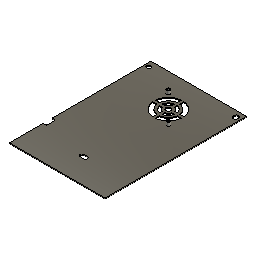
Ender 3 mainboard cover no-fan v10 (Autodesk Fusion 360 design; units mm, degrees)
Autodesk Fusion 360 part; units mm, degrees
sketch "Sketch1" plane through (0, 0, 0) normal (0, 0, 1) x (1, 0, 0)
  line L0 (-57.2, 86.75) -> (56, 86.75)
  line L1 (56, 86.75) -> (56, -80.25)
  line L2 (56, -80.25) -> (-57.2, -80.25)
  line L3 (-57.2, -80.25) -> (-57.2, 86.75)
  circle A0 centre (-52.2, 79.25) radius 2
  line L4 (48, 80) -> (48, 78.5)
  arc A1 (48, 78.5) -> (52, 78.5) centre (50, 78.5) ccw
  line L5 (52, 78.5) -> (52, 80)
  arc A2 (52, 80) -> (48, 80) centre (50, 80) ccw
  line L6 (50, 80) -> (50, 78.5) construction
  line L7 (-1.25, -51.95) -> (2.95, -51.95)
  arc A3 (2.95, -51.95) -> (2.95, -48.45) centre (2.95, -50.2) ccw
  line L8 (2.95, -48.45) -> (-1.25, -48.45)
  arc A4 (-1.25, -48.45) -> (-1.25, -51.95) centre (-1.25, -50.2) ccw
  line L9 (-3, -50.2) -> (4.7, -50.2) construction
  line L10 (-57.2, -30.05) -> (-53.2, -30.05)
  line L11 (-53.2, -30.05) -> (-53.2, -39.95)
  line L12 (-53.2, -39.95) -> (-57.2, -39.95)
  line L13 (-57.2, -39.95) -> (-57.2, -30.05)
  dimension "d1" = 113.2
  dimension "d2" = 167
  dimension "d3" = 4
  dimension "d4" = 5
  dimension "d5" = 7.5
  dimension "d6" = 4
  dimension "d7" = 1.5
  dimension "d8" = 6
  dimension "d9" = 6.75
  dimension "d10" = 3.5
  dimension "d11" = 7.7
  dimension "d12" = 28.3
  dimension "d13" = 51.3
  dimension "d14" = 9.9
  dimension "d15" = 4
  dimension "d16" = 40.3
  constraint horizontal L0
  constraint vertical L1
  constraint horizontal L2
  constraint vertical L3
  constraint tangent L4 A1
  constraint tangent A1 L5
  constraint parallel L4 L5
  constraint tangent L5 A2
  constraint tangent L4 A2
  constraint vertical L6
  constraint tangent L7 A3
  constraint tangent A3 L8
  constraint parallel L7 L8
  constraint tangent L8 A4
  constraint tangent L7 A4
  constraint midpoint A4 L9.start
  constraint midpoint A3 L9.end
  constraint horizontal L9
  constraint horizontal L10
  constraint vertical L11
  constraint horizontal L12
  constraint vertical L13
  constraint coincident L3 L10.start
  measures "d1" distance of L0.start L0.end
  measures "d2" distance of L0.start L2.end
  measures "d3" diameter of A0
  measures "d4" distance of L3 A0.centre
  measures "d5" distance of L0 A0.centre
  measures "d6" diameter of A1
  measures "d7" distance of A2.centre A1.centre
  measures "d8" distance of L1 A1.centre
  measures "d9" distance of L0 A2.centre
  measures "d10" diameter of A3
  measures "d11" distance of L9.start L9.end
  measures "d12" distance of L2 L7
  measures "d13" distance of L1 L9.end
  measures "d14" distance of L10.start L12.end
  measures "d15" distance of L10.start L10.end
  measures "d16" distance of L2 L12
  measures "d47" distance of L0.start
extrude "Extrude1" add sketch "Sketch1" along normal blind 1 contours L0 L1 L2 L3 L10 L11 L12
sketch "Sketch4" plane through (0, 0, 1) normal (0, 0, 1) x (-1, 0, 0)
  arc A0 (-52, -80) -> (-48, -80) centre (-50, -80) ccw
  line L0 (-52, -80) -> (-52, -78.5)
  arc A1 (-48, -78.5) -> (-52, -78.5) centre (-50, -78.5) ccw
  line L1 (-48, -78.5) -> (-48, -80)
  arc A2 (1.25, 48.45) -> (1.25, 51.95) centre (1.25, 50.2) ccw
  line L2 (1.25, 48.45) -> (-2.95, 48.45)
  arc A3 (-2.95, 51.95) -> (-2.95, 48.45) centre (-2.95, 50.2) ccw
  line L3 (-2.95, 51.95) -> (1.25, 51.95)
  circle A4 centre (52.2, -79.25) radius 2
  line L4 (57.2, 30.05) -> (53.2, 30.05)
  line L5 (53.2, 30.05) -> (53.2, 39.95)
  line L6 (53.2, 39.95) -> (57.2, 39.95)
  line L7 (57.2, 39.95) -> (57.2, 80.25)
  line L8 (57.2, 80.25) -> (-56, 80.25)
  line L9 (-56, 80.25) -> (-56, -86.75)
  line L10 (-56, -86.75) -> (57.2, -86.75)
  line L11 (57.2, -86.75) -> (57.2, 30.05)
  circle A5 centre (-2.375, -47.675) radius 16.875
  circle A6 centre (-2.375, -47.675) radius 12
  circle A7 centre (-2.375, -47.675) radius 9
  circle A8 centre (-2.375, -47.675) radius 6
  circle A9 centre (-2.375, -47.675) radius 3
  line L12 (-3.875, -66.4009) -> (-0.875, -66.4009)
  line L13 (-0.875, -66.4009) -> (-0.875, -28.9491)
  line L14 (-0.875, -28.9491) -> (-3.875, -28.9491)
  line L15 (-3.875, -28.9491) -> (-3.875, -66.4009)
  line L16 (-3.875, -66.4009) -> (-0.875, -28.9491) construction
  line L17 (-0.875, -66.4009) -> (-3.875, -28.9491) construction
  line L18 (-24.5082, -46.175) -> (19.7582, -46.175)
  line L19 (19.7582, -46.175) -> (19.7582, -49.175)
  line L20 (19.7582, -49.175) -> (-24.5082, -49.175)
  line L21 (-24.5082, -49.175) -> (-24.5082, -46.175)
  line L22 (-24.5082, -46.175) -> (19.7582, -49.175) construction
  line L23 (19.7582, -46.175) -> (-24.5082, -49.175) construction
  point P0 (-2.375, -47.675)
  point P1 (-2.375, -47.675)
  dimension "d42" = 33.75
  dimension "d43" = 24
  dimension "d44" = 18
  dimension "d45" = 12
  dimension "d46" = 6
  dimension "d47" = 3
  dimension "d48" = 3
  dimension "d59" = 39.075
  dimension "d60" = 53.625
  constraint concentric A5 A6
  constraint concentric A5 A7
  constraint concentric A6 A8
  constraint concentric A8 A9
  constraint perpendicular L12 L13
  constraint parallel L12 L14
  constraint parallel L13 L15
  constraint horizontal L12
  constraint coincident L16 P1
  constraint coincident L17 P1
  constraint coincident P1 P0
  constraint perpendicular L18 L19
  constraint parallel L18 L20
  constraint parallel L19 L21
  constraint horizontal L18
  constraint coincident L22 P1
  constraint coincident L23 P1
  measures "d42" diameter of A5
  measures "d43" diameter of A6
  measures "d44" diameter of A7
  measures "d45" diameter of A8
  measures "d46" diameter of A9
  measures "d47" distance of L13.end L14.end
  measures "d48" distance of L18.end L19.end
  measures "d59" distance of L10 P1
  measures "d60" distance of L9 P1
extrude "Extrude4" cut sketch "Sketch4" against normal through all contours A5 A6 L13 L18 | A5 A6 L13 L20 | A5 A6 L15 L18 | A7 A8 L13 L18 | A5 A6 L15 L20 | A7 A8 L13 L20 | A7 A8 L15 L18 | A9 L13 L18 | A9 L13 L18 L20 | A7 A8 L15 L20 | A9 L13 L20 | A9 L13 L15 L18 | L13 L15 L18 L20 | A9 L13 L15 L20 | A9 L15 L18 | A9 L15 L18 L20 | A9 L15 L20
sketch "Sketch5" plane through (0, 0, 1) normal (0, 0, 1) x (-1, 0, 0)
  arc A0 (-0.875, -59.5809) -> (9.5309, -49.175) centre (-2.375, -47.675) ccw
  line L0 (9.5309, -49.175) -> (14.4332, -49.175)
  arc A1 (-0.875, -64.4832) -> (14.4332, -49.175) centre (-2.375, -47.675) ccw
  line L1 (-0.875, -64.4832) -> (-0.875, -59.5809)
  arc A2 (-14.2809, -49.175) -> (-3.875, -59.5809) centre (-2.375, -47.675) ccw
  line L2 (-3.875, -59.5809) -> (-3.875, -64.4832)
  arc A3 (-19.1832, -49.175) -> (-3.875, -64.4832) centre (-2.375, -47.675) ccw
  line L3 (-19.1832, -49.175) -> (-14.2809, -49.175)
  arc A4 (-3.875, -35.7691) -> (-14.2809, -46.175) centre (-2.375, -47.675) ccw
  line L4 (-14.2809, -46.175) -> (-19.1832, -46.175)
  arc A5 (-3.875, -30.8668) -> (-19.1832, -46.175) centre (-2.375, -47.675) ccw
  line L5 (-3.875, -30.8668) -> (-3.875, -35.7691)
  arc A6 (-0.875, -53.4845) -> (3.4345, -49.175) centre (-2.375, -47.675) ccw
  line L6 (3.4345, -49.175) -> (6.4991, -49.175)
  arc A7 (-0.875, -56.5491) -> (6.4991, -49.175) centre (-2.375, -47.675) ccw
  line L7 (-0.875, -56.5491) -> (-0.875, -53.4845)
  arc A8 (-3.875, -41.8655) -> (-8.1845, -46.175) centre (-2.375, -47.675) ccw
  line L8 (-8.1845, -46.175) -> (-11.2491, -46.175)
  arc A9 (-3.875, -38.8009) -> (-11.2491, -46.175) centre (-2.375, -47.675) ccw
  line L9 (-3.875, -38.8009) -> (-3.875, -41.8655)
  arc A10 (3.4345, -46.175) -> (-0.875, -41.8655) centre (-2.375, -47.675) ccw
  line L10 (-0.875, -41.8655) -> (-0.875, -38.8009)
  arc A11 (6.4991, -46.175) -> (-0.875, -38.8009) centre (-2.375, -47.675) ccw
  line L11 (6.4991, -46.175) -> (3.4345, -46.175)
  circle A12 centre (-2.375, -47.675) radius 3
  arc A13 (9.5309, -46.175) -> (-0.875, -35.7691) centre (-2.375, -47.675) ccw
  line L12 (-0.875, -35.7691) -> (-0.875, -30.8668)
  arc A14 (14.4332, -46.175) -> (-0.875, -30.8668) centre (-2.375, -47.675) ccw
  line L13 (14.4332, -46.175) -> (9.5309, -46.175)
  arc A15 (-8.1845, -49.175) -> (-3.875, -53.4845) centre (-2.375, -47.675) ccw
  line L14 (-3.875, -53.4845) -> (-3.875, -56.5491)
  arc A16 (-11.2491, -49.175) -> (-3.875, -56.5491) centre (-2.375, -47.675) ccw
  line L15 (-11.2491, -49.175) -> (-8.1845, -49.175)
  arc A17 (-52, -80) -> (-48, -80) centre (-50, -80) ccw
  line L16 (-52, -80) -> (-52, -78.5)
  arc A18 (-48, -78.5) -> (-52, -78.5) centre (-50, -78.5) ccw
  line L17 (-48, -78.5) -> (-48, -80)
  arc A19 (1.25, 48.45) -> (1.25, 51.95) centre (1.25, 50.2) ccw
  line L18 (1.25, 48.45) -> (-2.95, 48.45)
  arc A20 (-2.95, 51.95) -> (-2.95, 48.45) centre (-2.95, 50.2) ccw
  line L19 (-2.95, 51.95) -> (1.25, 51.95)
  circle A21 centre (52.2, -79.25) radius 2
  line L20 (57.2, 30.05) -> (53.2, 30.05)
  line L21 (53.2, 30.05) -> (53.2, 39.95)
  line L22 (53.2, 39.95) -> (57.2, 39.95)
  line L23 (57.2, 39.95) -> (57.2, 80.25)
  line L24 (57.2, 80.25) -> (-56, 80.25)
  line L25 (-56, 80.25) -> (-56, -86.75)
  line L26 (-56, -86.75) -> (57.2, -86.75)
  line L27 (57.2, -86.75) -> (57.2, 30.05)
  circle A22 centre (13.6056, -63.6556) radius 2.05
  circle A23 centre (-18.3556, -31.6944) radius 2.05
  line L28 (13.6056, -63.6556) -> (-18.3556, -31.6944) construction
  circle A24 centre (13.6056, -63.6556) radius 1.25
  circle A25 centre (-18.3556, -31.6944) radius 1.25
  dimension "d51" = 4.1
  dimension "d52" = 4.1
  dimension "d53" = 45.2
  dimension "d54" = 45
  dimension "d55" = 2.5
  dimension "d56" = 2.5
  constraint coincident A22.centre L28.start
  constraint coincident A23.centre L28.end
  constraint coincident A0.centre L28
  constraint midpoint A0.centre L28
  measures "d51" diameter of A22
  measures "d52" diameter of A23
  measures "d53" distance of A22.centre A23.centre
  measures "d54" angle of L4 L28
  measures "d55" diameter of A24
  measures "d56" diameter of A25
extrude "Extrude5" add sketch "Sketch5" along normal blind 4.2 contours A22 | A23
fillet "Fillet4" radius 1 8 edges at (56, -80.25, 0.5) (-57.2, -80.25, 0.5) (-57.2, -39.95, 0.5) (-53.2, -39.95, 0.5) (-57.2, -30.05, 0.5) (-53.2, -30.05, 0.5) (-57.2, 86.75, 0.5) (56, 86.75, 0.5)
fillet "Fillet5" radius 0.5 50 edges at (-56.9071, -79.9571, 1) (-0.6, -80.25, 1) (55.7071, -79.9571, 1) (56, 3.25, 1) (55.7071, 86.4571, 1) (-0.6, 86.75, 1) (-56.9071, 86.4571, 1) (-57.2, 28.35, 1) (-56.9071, -29.7571, 1) (-55.2, -30.05, 1) (-53.4929, -30.3429, 1) (-53.2, -35, 1) (-53.4929, -39.6571, 1) (-55.2, -39.95, 1) (-56.9071, -40.2429, 1) (-57.2, -60.1, 1) (-56.9071, -40.2429, 0) (-55.2, -39.95, 0) (-53.4929, -39.6571, 0) (-53.2, -35, 0) (-53.4929, -30.3429, 0) (-55.2, -30.05, 0) (-56.9071, -29.7571, 0) (-57.2, 28.35, 0) (-56.9071, 86.4571, 0) (-0.6, 86.75, 0) (55.7071, 86.4571, 0) (56, 3.25, 0) (55.7071, -79.9571, 0) (-0.6, -80.25, 0) (-56.9071, -79.9571, 0) (-57.2, -60.1, 0) (-3, -50.2, 1) (0.85, -48.45, 1) (4.7, -50.2, 1) (0.85, -51.95, 1) (-3, -50.2, 0) (0.85, -48.45, 0) (4.7, -50.2, 0) (0.85, -51.95, 0) (-54.0647, 79.9732, 1) (-54.0647, 79.9732, 0) (50, 82, 1) (52, 79.25, 1) (50, 76.5, 1) (48, 79.25, 1) (50, 82, 0) (52, 79.25, 0) (50, 76.5, 0) (48, 79.25, 0)
chamfer "Chamfer1" distance 0.5 angle 45 2 edges at (-12.4402, 63.2036, 5.2) (19.521, 31.2424, 5.2)
equation "d59 = 22.2 mm + ( 33.75 / 2 ) * 1 mm"
equation "d60 = 36.75 mm + ( 33.75 / 2 ) * 1 mm"
